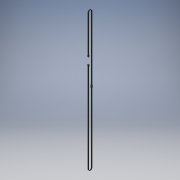
# Autodesk Inventor part: second stage belt 2
Saved by Autodesk Inventor 2017 SP1 (Build 210196100, 196)
## iProperties
Created: 2018-01-21
Part Number: second stage belt 2
Material: Rubber
Document SubType Name: Modeling
Designer: Ben
Density: 0.93 g/cm^3
Appearance: Rubber - Black
Mass: 35.9399 g
Surface Area: 567.611 cm^2
Volume: 38.645 cm^3
Author: Ben
Autodesk Inventor part; units mm, degrees
ref_plane "YZ Plane" through (0, 0, 0) normal (1, 0, 0) x (0, 1, 0)
ref_plane "XZ Plane" through (0, 0, 0) normal (0, 1, 0) x (-1, 0, 0)
ref_plane "XY Plane" through (0, 0, 0) normal (0, 0, 1) x (1, 0, 0)
sketch "Sketch1" plane through (0, 0, 0) normal (1, 0, 0) x (0, 1, 0)
  line L0 (562.6735, 0) -> (251.3795, 0)
  arc A0 (562.6735, -28.575) -> (562.6735, 0) centre (562.6735, -14.2875) ccw
  line L1 (562.6735, -28.575) -> (17.9029, -28.575)
  arc A1 (-616.204, 0) -> (-616.204, -28.575) centre (-616.204, -14.2875) ccw
  line L2 (-616.204, -28.575) -> (-17.9029, -28.575)
  line L3 (17.9029, -30.1625) -> (562.6735, -30.1625)
  arc A2 (562.6735, -30.1625) -> (562.6735, 1.5875) centre (562.6735, -14.2875) ccw
  line L4 (562.6735, 1.5875) -> (251.3795, 1.5875)
  arc A3 (-616.204, 1.5875) -> (-616.204, -30.1625) centre (-616.204, -14.2875) ccw
  line L5 (-616.204, -30.1625) -> (-17.9029, -30.1625)
  arc A4 (0.8555, -23.8265) -> (-0.8555, -23.8265) centre (0, -28.5115) ccw
  arc A5 (17.9029, -28.575) -> (16.7623, -28.6783) centre (17.9029, -34.925) ccw
  line L6 (16.7623, -28.6783) -> (4.0623, -30.9972)
  arc A6 (17.9029, -30.1625) -> (17.0475, -30.24) centre (17.9029, -34.925) ccw
  line L7 (17.0475, -30.24) -> (0.8555, -33.1965)
  arc A7 (16.7623, -28.3447) -> (17.9029, -28.448) centre (17.9029, -22.098) ccw
  line L8 (17.9029, -28.448) -> (30.6029, -28.448)
  line L9 (16.7623, -28.3447) -> (4.0623, -26.0258)
  line L10 (17.9029, -28.448) -> (17.9029, -28.575) construction
  line L11 (30.6029, -28.448) -> (30.6029, -26.8605)
  line L12 (30.6029, -26.8605) -> (17.9029, -26.8605)
  arc A8 (17.0475, -26.783) -> (17.9029, -26.8605) centre (17.9029, -22.098) ccw
  line L13 (17.0475, -26.783) -> (0.8555, -23.8265)
  arc A9 (-17.0475, -30.24) -> (-17.9029, -30.1625) centre (-17.9029, -34.925) ccw
  arc A10 (-16.7623, -28.6783) -> (-17.9029, -28.575) centre (-17.9029, -34.925) ccw
  line L14 (-16.7623, -28.6783) -> (-4.0623, -30.9972)
  arc A11 (-0.8555, -33.1965) -> (0.8555, -33.1965) centre (0, -28.5115) ccw
  line L15 (-0.8555, -33.1965) -> (-17.0475, -30.24)
  arc A12 (-17.9029, -28.448) -> (-16.7623, -28.3447) centre (-17.9029, -22.098) ccw
  line L16 (-17.9029, -28.575) -> (-17.9029, -28.448) construction
  line L17 (-17.9029, -28.448) -> (-30.6029, -28.448)
  line L18 (-30.6029, -28.448) -> (-30.6029, -26.8605)
  line L19 (-30.6029, -26.8605) -> (-17.9029, -26.8605)
  arc A13 (-17.9029, -26.8605) -> (-17.0475, -26.783) centre (-17.9029, -22.098) ccw
  line L20 (-17.0475, -26.783) -> (-0.8555, -23.8265)
  line L21 (162.958, 0) -> (-616.204, 0)
  line L22 (162.958, 1.5875) -> (-616.204, 1.5875)
  arc A14 (237.2515, 3.0937) -> (237.2221, -3.1003) centre (236.5375, 0) ccw
  arc A15 (249.9515, 0.1626) -> (251.3795, 0) centre (251.3795, 6.35) ccw
  line L23 (249.9515, 0.1626) -> (237.2515, 3.0937)
  line L24 (250.3085, 1.7095) -> (237.6085, 4.6405)
  arc A16 (237.6085, 4.6405) -> (237.5644, -4.6505) centre (236.5375, 0) ccw
  arc A17 (4.0623, -30.9972) -> (4.0623, -26.0258) centre (0, -28.5115) ccw
  line L25 (-4.0623, -26.0258) -> (-16.7623, -28.3447)
  arc A18 (0.8555, -23.8265) -> (-0.8555, -23.8265) centre (0, -28.5115) ccw
  arc A19 (-4.0623, -26.0258) -> (-4.0623, -30.9972) centre (0, -28.5115) ccw
  arc A20 (-0.8555, -33.1965) -> (0.8555, -33.1965) centre (0, -28.5115) ccw
  circle A21 centre (0, -28.5115) radius 3.175
  arc A22 (250.3085, 1.7095) -> (251.3795, 1.5875) centre (251.3795, 6.35) ccw
  arc A23 (251.3795, -0.127) -> (250.0102, -0.2764) centre (251.3795, -6.477) ccw
  arc A24 (251.3795, -1.7145) -> (250.3525, -1.8265) centre (251.3795, -6.477) ccw
  line L26 (251.3795, -0.127) -> (264.0795, -0.127)
  line L27 (264.0795, -0.127) -> (264.0795, -1.7145)
  line L28 (264.0795, -1.7145) -> (251.3795, -1.7145)
  line L29 (250.0102, -0.2764) -> (237.2221, -3.1003)
  line L30 (237.5644, -4.6505) -> (250.3525, -1.8265)
  line L31 (251.3795, 0) -> (251.3795, -0.127) construction
  arc A25 (177.1154, -3.1003) -> (177.086, 3.0937) centre (177.8, 0) ccw
  arc A26 (176.7731, -4.6505) -> (176.729, 4.6405) centre (177.8, 0) ccw
  arc A27 (162.958, 0) -> (164.386, 0.1626) centre (162.958, 6.35) ccw
  arc A28 (162.958, 1.5875) -> (164.029, 1.7095) centre (162.958, 6.35) ccw
  line L32 (177.086, 3.0937) -> (164.386, 0.1626)
  line L33 (176.729, 4.6405) -> (164.029, 1.7095)
  arc A29 (164.3273, -0.2764) -> (162.958, -0.127) centre (162.958, -6.477) ccw
  arc A30 (163.985, -1.8265) -> (162.958, -1.7145) centre (162.958, -6.477) ccw
  line L34 (162.958, -0.127) -> (150.258, -0.127)
  line L35 (150.258, -0.127) -> (150.258, -1.7145)
  line L36 (150.258, -1.7145) -> (162.958, -1.7145)
  line L37 (177.1154, -3.1003) -> (164.3273, -0.2764)
  line L38 (176.7731, -4.6505) -> (163.985, -1.8265)
  line L39 (162.958, -0.127) -> (162.958, 0) construction
  line L40 (0, 0) -> (0, -28.5115) construction
  dimension "d1" = 14.2875
  dimension "d5" = 1.5875
  dimension "d7" = 6.35
  dimension "d9" = 12.7
  dimension "d10" = 0.127
  dimension "d11" = 6.35
  dimension "d13" = 0.127
  dimension "d14" = 12.7
  dimension "d15" = 1178.8775
  dimension "d20" = 6.35
  dimension "d22" = 12.7
  dimension "d23" = 12.7
  dimension "d24" = 0.127
  dimension "d25" = 12.7
  dimension "d27" = 58.7375
  dimension "d30" = 177.8
  dimension "d31" = 616.204
  dimension "d32" = 14.2875
  constraints: 82 end point, 61 point on circle, 56 tangent, 31 centre point, 12 coincident, 9 horizontal, 9 parallel, 8 equal radius, 7 equal length, 6 perpendicular, 5 vertical, 3 point on line, 2 collinear, 1 concentric, 1 line through centre, 2 other
  measures "d1" radius of A0
  measures "d5" distance between parallel lines of L4 L0
  measures "d7" radius of A5
  measures "d9" distance of L8.start L8.end
  measures "d10" distance between parallel lines of L8 L1
  measures "d11" radius of A10
  measures "d13" distance of L2.end L16.end
  measures "d14" distance of L16.end L17.end
  measures "d15" distance of A1.centre A0.centre
  measures "d20" diameter of A21
  measures "d22" horizontal distance of L9.start L9.end
  measures "d23" horizontal distance of L23.start L23.end
  measures "d24" distance between parallel lines of L26 L0
  measures "d25" distance of L27.end L28.end
  measures "d27" distance of A14.centre A25.centre
  measures "d30" distance from line of L40 A25.centre
  measures "d31" distance from line of A1.centre L40
  measures "d32" radius of A1
extrude "Extrusion1" add sketch "Sketch1" along normal mid plane 9.525
body "Solid1"
